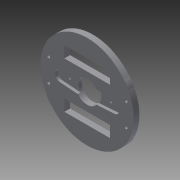
# Autodesk Inventor part: kinectUchyt
Saved by Autodesk Inventor 2016 (Build 200138000, 138)
## iProperties
Created: 2015-11-06
Part Number: kinectUchyt
Material: Generic
Document SubType Name: Modeling
Designer: Jufo
Density: 1 g/cm^3
Appearance: Default
Author: Jufo
Autodesk Inventor part; units mm, degrees
ref_plane "YZ Plane" through (0, 0, 0) normal (1, 0, 0) x (0, 1, 0)
ref_plane "XZ Plane" through (0, 0, 0) normal (0, 1, 0) x (-1, 0, 0)
ref_plane "XY Plane" through (0, 0, 0) normal (0, 0, 1) x (1, 0, 0)
sketch "Sketch3" plane through (0, 0, 0) normal (0, 1, 0) x (-1, 0, 0)
  line L0 (-17.2768, 43.3118) -> (-17.2768, 17.2768)
  line L1 (57.2818, 17.2768) -> (57.2818, 43.3118)
  line L2 (40.005, 60.5886) -> (0, 60.5886)
  line L3 (0, 0) -> (40.005, 0)
  arc A0 (0, 60.5886) -> (-17.2768, 43.3118) centre (0, 43.3118) ccw
  arc A1 (57.2818, 43.3118) -> (40.005, 60.5886) centre (40.005, 43.3118) ccw
  arc A2 (57.2818, 43.3118) -> (40.005, 60.5886) centre (40.005, 43.3118) ccw
  arc A3 (40.005, 0) -> (57.2818, 17.2768) centre (40.005, 17.2768) ccw
  arc A4 (40.005, 0) -> (57.2818, 17.2768) centre (40.005, 17.2768) ccw
  arc A5 (-17.2768, 17.2768) -> (0, 0) centre (0, 17.2768) ccw
  line L4 (-17.2768, 43.3118) -> (-17.2768, 17.2768)
  line L5 (-17.2768, 17.2768) -> (-23.495, 17.2768)
  line L6 (0, 60.5886) -> (40.005, 60.5886)
  line L7 (57.2818, 43.3118) -> (57.2818, 17.2768)
  line L8 (-13.9768, 30.2943) -> (-13.9768, 40.2943)
  circle A6 centre (-13.9768, 40.2943) radius 1.5
  line L9 (-17.2768, 30.2943) -> (28.6458, 30.2943)
  line L10 (20.0025, 60.5886) -> (20.0025, 11.8486)
  circle A7 centre (-13.9768, 20.2943) radius 1.5
  circle A8 centre (54.0232, 40.2943) radius 1.5
  circle A9 centre (54.0232, 20.2943) radius 1.5
  line L11 (20.0025, 30.2943) -> (2.0025, 30.2943)
  circle A10 centre (2.0025, 30.2943) radius 1
  circle A11 centre (38.0025, 30.2943) radius 1
  line L12 (40.005, 5) -> (0, 5)
  line L13 (0, 5) -> (0, 15)
  line L14 (0, 15) -> (40.005, 15)
  line L15 (40.005, 15) -> (40.005, 5)
  line L16 (40.005, 55.5886) -> (0, 55.5886)
  line L17 (0, 55.5886) -> (0, 45.5886)
  line L18 (0, 45.5886) -> (40.005, 45.5886)
  line L19 (40.005, 45.5886) -> (40.005, 55.5886)
  circle A12 centre (20.0025, 30.2943) radius 40.9246
  dimension "d4" = 74.5586
  dimension "d5" = 60.5886
  dimension "d7" = 10
  dimension "d8" = 3
  dimension "d11" = 20
  dimension "d14" = 68
  dimension "d17" = 3.3
  dimension "d18" = 18
  dimension "d19" = 2
  dimension "d21" = 5
  dimension "d22" = 10
  constraints: 40 end point, 15 point on circle, 13 centre point, 5 symmetric about line, 4 perpendicular, 4 tangent, 3 vertical, 2 coincident, 2 horizontal, 2 midpoint, 1 collinear, 1 point on line, 7 other
  measures "d4" distance between parallel lines of L0 L1
  measures "d5" distance between parallel lines of L2 L3
  measures "d7" distance of L8.start L8.end
  measures "d8" diameter of A6
  measures "d11" distance of A6.centre A7.centre
  measures "d14" distance of A6.centre A8.centre
  measures "d17" distance from line of L0 A6.centre
  measures "d18" distance of L11.start L11.end
  measures "d19" diameter of A10
  measures "d21" distance of A4.start L12.start
  measures "d22" distance of L12.end L13.end
extrude "Extrusion4" add sketch "Sketch3" along normal blind 5 contours A0 A12 L2 L10 L16 L17 L18 L9 A10 L0 | L0 L5 A12 A0 | L9 A10 L10 L18 L19 L16 L2 A1 A12 L1 A3 L3 A5 L0 | A0 A12 | A5 A12 L5 | A12 A1 L2 A0 | A12 A5 | A1 A12 | A5 L3 A3 A12 | A12 A3 L1 A1 | A12 A3
sketch "Sketch5" plane through (0, 0, 0) normal (0, -1, 0) x (1, 0, 0)
  circle A0 centre (-20.0025, 30.2943) radius 6.5
  line L0 (-20.0025, 30.2943) -> (7.9975, 30.2943)
  line L1 (7.9975, 30.2943) -> (7.9975, 25.7943)
  line L2 (7.9975, 25.7943) -> (-20.0025, 23.7943)
  line L3 (7.9975, 30.2943) -> (7.9975, 34.7943)
  line L4 (7.9975, 34.7943) -> (-20.0025, 36.7943)
  line L5 (-20.0025, 20.7562) -> (-20.0025, 45.1513)
  line L6 (-48.0025, 30.2943) -> (-48.0025, 25.7943)
  line L7 (-48.0025, 25.7943) -> (-20.0025, 23.7943)
  line L8 (-48.0025, 30.2943) -> (-48.0025, 34.7943)
  line L9 (-48.0025, 34.7943) -> (-20.0025, 36.7943)
  point P0 (0, 0)
  dimension "d30" = 13
  dimension "d31" = 28
  dimension "d32" = 4.5
  dimension "d33" = 4.5
  constraints: 20 end point, 3 symmetric about line, 2 point on circle, 2 vertical, 1 centre point, 1 horizontal
  measures "d30" diameter of A0
  measures "d31" distance of L0.start L0.end
  measures "d32" distance of L0.end L1.end
  measures "d33" distance of L0.end L3.end
extrude "Extrusion5" cut sketch "Sketch5" against normal blind 2.5
fillet "Fillet1" radius 4 4 edges at (7.9975, 1.25, 25.7943) (-48.0025, 1.25, 34.7943) (7.9975, 1.25, 34.7943) (-48.0025, 1.25, 25.7943)
sketch "Sketch7" plane through (0, 5, 0) normal (0, 1, 0) x (1, 0, 0)
  circle A0 centre (-20.0025, -30.2943) radius 10
  point P0 (0, 0)
  dimension "d39" = 20
  constraints: 1 centre point
  measures "d39" diameter of A0
extrude "Extrusion6" cut sketch "Sketch7" against normal blind 5
body "Solid4"
